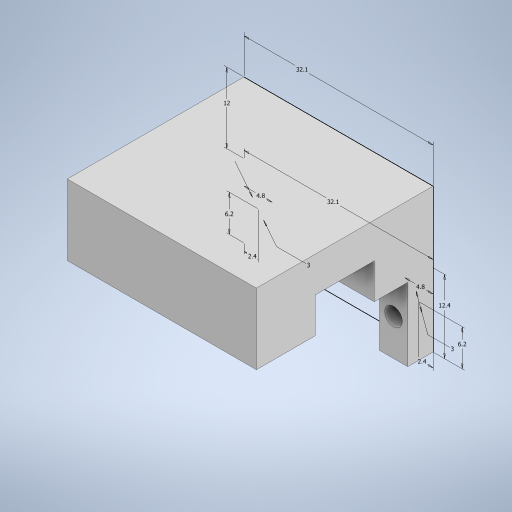
# Autodesk Inventor part: 固定塊
Saved by Autodesk Inventor 2024 (Build 280153000, 153)
## iProperties
Created: 2024-04-21
Part Number: 固定塊
Material: 一般
Document SubType Name: Modeling
Designer: rumse
Density: 1 g/cm^3
Appearance: 預設
Author: rumse
Autodesk Inventor part; units mm, degrees
ref_plane "YZ Plane" through (0, 0, 0) normal (1, 0, 0) x (0, 1, 0)
ref_plane "XZ Plane" through (0, 0, 0) normal (0, 1, 0) x (-1, 0, 0)
ref_plane "XY Plane" through (0, 0, 0) normal (0, 0, 1) x (1, 0, 0)
sketch "草圖1" plane through (0, 0, 0) normal (0, 0, 1) x (1, 0, 0)
  line L0 (0, 0) -> (32.1, 0)
  line L1 (32.1, 0) -> (32.1, 12.4)
  line L2 (32.1, 12.4) -> (0, 12.4)
  line L3 (0, 12.4) -> (0, 0)
  line L4 (4.8, 12.4) -> (4.8, 0)
  line L5 (27.3, 12.4) -> (27.3, 0)
  line L6 (32.1, 12.4) -> (0, 12.4)
  line L7 (0, 12.4) -> (0, 24.4)
  line L8 (0, 24.4) -> (32.1, 24.4)
  line L9 (32.1, 24.4) -> (32.1, 12.4)
  circle A0 centre (2.4, 6.2) radius 1.5
  circle A1 centre (29.7, 6.2) radius 1.5
  point P0 (0, 12.4)
  dimension "d0" = 12.4
  dimension "d1" = 32.1
  dimension "d2" = 4.8
  dimension "d3" = 4.8
  dimension "d6" = 12
  dimension "d7" = 32.1
  dimension "d14" = 6.2
  dimension "d15" = 6.2
  dimension "d16" = 2.4
  dimension "d17" = 2.4
  dimension "d18" = 3
  dimension "d19" = 3
  constraints: 20 end point, 4 parallel, 4 perpendicular, 4 point on line, 2 centre point, 2 horizontal
  measures "d0" distance of L0.end L1.end
  measures "d1" distance of L1.end L2.end
  measures "d2" distance between parallel lines of L4 L3
  measures "d3" distance between parallel lines of L1 L5
  measures "d6" distance of L6.end L7.end
  measures "d7" distance of L7.end L8.end
  measures "d14" vertical distance of L0.start A0.centre
  measures "d15" distance from line of L0 A1.centre
  measures "d16" horizontal distance of L0.end A1.centre
  measures "d17" horizontal distance of L0.start A0.centre
  measures "d18" diameter of A0
  measures "d19" diameter of A1
extrude "擠出1" add sketch "草圖1" along normal blind 4.3 contours L3 L2 L4 L0 | L5 L2 L1 L0 | A0 | A1
extrude "擠出2" add sketch "草圖1" along normal blind 10 contours L7 L8 L9 L2
sketch "草圖2" plane through (0, 0, 10) normal (0, 0, 1) x (1, 0, 0)
  line L0 (32.1, 24.4) -> (0, 24.4) projected
  line L1 (0, 24.4) -> (0, 12.4) projected
  line L2 (0, 12.4) -> (32.1, 12.4) projected
  line L3 (32.1, 12.4) -> (32.1, 24.4) projected
  line L4 (0, 24.4) -> (32.1, 24.4)
  line L5 (32.1, 24.4) -> (32.1, 18.4)
  line L6 (32.1, 18.4) -> (0, 18.4)
  line L7 (0, 18.4) -> (0, 24.4)
  point P0 (0, 0)
  point P1 (0, 18.4)
  constraints: 8 end point, 2 parallel, 1 horizontal, 1 midpoint, 1 perpendicular
extrude "擠出3" add sketch "草圖2" along normal blind 10 contours L3 L6 L1 L0
sketch "草圖3" plane through (0, 0, 20) normal (0, 0, 1) x (1, 0, 0)
  line L0 (32.1, 18.4) -> (32.1, 24.4) projected
  line L1 (32.1, 24.4) -> (0, 24.4) projected
  line L2 (0, 24.4) -> (0, 18.4) projected
  line L3 (0, 18.4) -> (32.1, 18.4) projected
  line L4 (32.1, 18.4) -> (0, 18.4) projected
  line L5 (0, 18.4) -> (0, 12.4) projected
  line L6 (0, 12.4) -> (32.1, 12.4) projected
  line L7 (32.1, 12.4) -> (32.1, 18.4) projected
  line L8 (0, 12.4) -> (32.1, 12.4)
  line L9 (32.1, 12.4) -> (32.1, 24.4)
  line L10 (32.1, 24.4) -> (0, 24.4)
  line L11 (0, 24.4) -> (0, 12.4)
  point P0 (0, 0)
  constraints: 8 end point, 2 parallel, 1 horizontal, 1 perpendicular
extrude "擠出4" add sketch "草圖3" along normal blind 10
extrude "擠出5" cut sketch "草圖1" along normal through all contours A0 | A1
